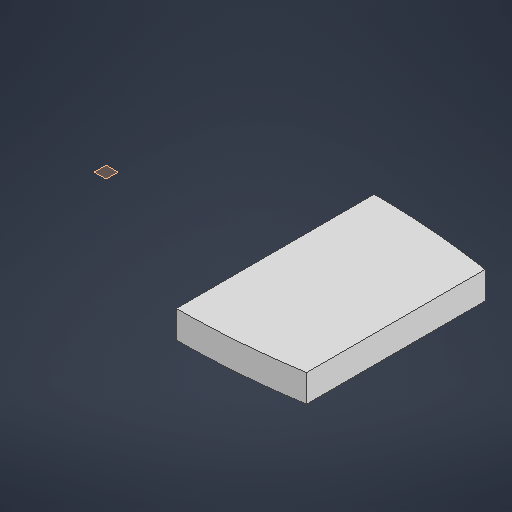
# Autodesk Inventor part: Soporte muñeca
Saved by Autodesk Inventor 2027 (Build 310192060, 192F)
## iProperties
Created: 2026-05-27
Part Number: Soporte muñeca
Material: Genérico
Document SubType Name: Modeling
Designer: nvaro
Density: 1 g/cm^3
Appearance: Valor por defecto
Author: nvaro
Autodesk Inventor part; units mm, degrees
ref_plane "YZ Plane" through (0, 0, 0) normal (1, 0, 0) x (0, 1, 0)
ref_plane "XZ Plane" through (0, 0, 0) normal (0, 1, 0) x (-1, 0, 0)
ref_plane "XY Plane" through (0, 0, 0) normal (0, 0, 1) x (1, 0, 0)
ref_plane "Plano de trabajo1" through (0, 50, 0) normal (0, 1, 0) x (1, 0, 0)
sketch "Boceto2" plane through (0, 50, 0) normal (0, 1, 0) x (1, 0, 0)
  line L0 (500.6332, -134.0891) -> (500.6333, 192.4676)
  line L1 (280.0654, 210.0497) -> (280.0653, -151.6711)
  line L2 (280.0654, 210.0497) -> (390.3494, 210.0497) construction
  line L3 (390.3494, 210.0497) -> (500.6333, 192.4676) construction
  spline S0 degree 2 poles (280.0654, 210.0497) (390.3494, 210.0497) (500.6333, 192.4676) knots 1 1 1 2 2 2
  spline S1 degree 2 poles (280.0653, -151.6711) (390.3493, -151.6711) (500.6332, -134.0891) knots 1 1 1 2 2 2
  line L4 (280.0653, -151.6711) -> (390.3493, -151.6711) construction
  line L5 (390.3493, -151.6711) -> (500.6332, -134.0891) construction
  line L6 (-182.5078, -134.4984) -> (-182.5078, 209.4027) projected
  line L7 (-163.212, -134.4984) -> (-182.5078, -134.4984) projected
  line L8 (-182.5078, 209.4027) -> (-170.0243, 209.4027) projected
  arc A0 (158.2881, -64.7914) -> (141.8037, 119.3131) centre (-117.1057, 3.3405) ccw
  line L9 (280.0654, 86.9847) -> (280.0654, 119.3131)
  arc A1 (166.3277, 13.9754) -> (163.3188, 46.3037) centre (-97.2594, 5.7469) ccw
  point P0 (0, 0)
  point P1 (-85.0735, -155.8983)
  point P2 (120.8954, -149.1961)
  point P3 (0.0587, 221.333)
  point P4 (141.8037, 86.9847)
  point P5 (141.8037, -60.9345)
  constraints: 6 end point, 5 point on circle, 2 centre point, 1 parallel, 1 point on line, 13 other
extrude "Extrusión5" add sketch "Boceto2" against normal blind 50 contours S1 L1 S0 L0
